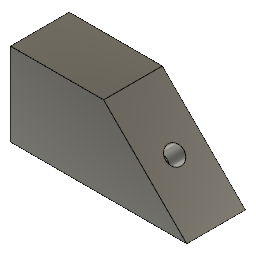
angled holder v2 (Autodesk Fusion 360 design; units mm, degrees)
Autodesk Fusion 360 part; units mm, degrees
sketch "holder body" plane through (0, 0, 0) normal (0, 0, 1) x (1, 0, 0)
  line L0 (0, 0) -> (30, 0)
  line L1 (30, 0) -> (15.8579, 14.1421)
  line L2 (15.8579, 14.1421) -> (0, 14.1421)
  line L3 (0, 14.1421) -> (0, 0)
  dimension "d1" = 20
  dimension "d2" = 45
  dimension "d3" = 30
  constraint coincident L0.start L3.end
  constraint horizontal L0
  constraint horizontal L2
  constraint perpendicular L2 L3
  measures "d1" distance of L0.end L1.end
  measures "d2" angle of L0 L1
  measures "d3" distance of L0.start L0.end
extrude "Extrude1" add sketch "holder body" along normal blind 10
move_body "Move1" bodies 1 to x (1, 0, 0) y (0, 0, 1) z (0, -1, 0) at (0, 0, 0)
sketch "hole for tube" plane through (15, 0, 15) normal (0.707107, 0, 0.707107) x (0, 1, 0)
  line L0 (0, -21.2132) -> (0, -1.2132)
  line L1 (0, -1.2132) -> (-10, -1.2132)
  line L2 (-10, -1.2132) -> (-10, -21.2132)
  line L3 (-10, -21.2132) -> (0, -21.2132)
  line L4 (-5, -1.2132) -> (-5, -21.2132) construction
  circle A0 centre (-5, -11.2132) radius 1.55
  dimension "d6" = 3.1
  constraint midpoint L1 L4.start
  constraint midpoint L3 L4.end
  constraint coincident L4 A0.centre
  constraint midpoint L4 A0.centre
  measures "d6" diameter of A0
extrude "Extrude2" cut sketch "hole for tube" against normal blind 4 contours A0
